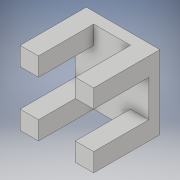
# Autodesk Inventor part: STand_1
Saved by Autodesk Inventor 2019 (Build 230136000, 136)
## iProperties
Created: 2020-02-20
Part Number: STand_1
Material: Generic
Document SubType Name: Modeling
Designer: Chirag
Density: 1 g/cm^3
Appearance: Default
Author: Chirag
Autodesk Inventor part; units mm, degrees
ref_plane "YZ Plane" through (0, 0, 0) normal (1, 0, 0) x (0, 1, 0)
ref_plane "XZ Plane" through (0, 0, 0) normal (0, 1, 0) x (-1, 0, 0)
ref_plane "XY Plane" through (0, 0, 0) normal (0, 0, 1) x (1, 0, 0)
sketch "Sketch1" plane through (0, 0, 0) normal (0, 0, 1) x (1, 0, 0)
  line L0 (0, 0) -> (0, -200)
  line L1 (0, -200) -> (200, -200)
  line L2 (200, -200) -> (200, 0)
  line L3 (200, 0) -> (0, 0)
  dimension "d0" = 200
  dimension "d1" = 200
  constraints: 8 end point, 2 parallel, 1 perpendicular, 1 vertical
  measures "d0" distance of L0.start L0.end
  measures "d1" distance of L1.end L0.end
extrude "Extrusion1" add sketch "Sketch1" along normal blind 30
sketch "Sketch2" plane through (0, 0, 30) normal (0, 0, 1) x (1, 0, 0)
  line L0 (0, 0) -> (0, -200) projected
  line L1 (0, 0) -> (0, -50)
  line L2 (0, -50) -> (50, -50)
  line L3 (50, -50) -> (50, 0)
  line L4 (50, 0) -> (0, 0)
  line L5 (200, -200) -> (200, 0) projected
  line L6 (200, 0) -> (200, -50)
  line L7 (200, -50) -> (150, -50)
  line L8 (150, -50) -> (150, 0)
  line L9 (150, 0) -> (200, 0)
  line L10 (0, -200) -> (0, -150)
  line L11 (0, -150) -> (50, -150)
  line L12 (50, -150) -> (50, -200)
  line L13 (50, -200) -> (0, -200)
  line L14 (200, -200) -> (200, -150)
  line L15 (200, -150) -> (150, -150)
  line L16 (150, -150) -> (150, -200)
  line L17 (150, -200) -> (200, -200)
  dimension "d4" = 50
  dimension "d5" = 50
  dimension "d6" = 50
  dimension "d7" = 50
  dimension "d8" = 50
  dimension "d9" = 50
  dimension "d10" = 50
  dimension "d11" = 50
  constraints: 32 end point, 8 parallel, 4 perpendicular, 4 point on line
  measures "d4" distance of L0.start L1.end
  measures "d5" distance of L2.end L1.end
  measures "d6" distance of L5.end L6.end
  measures "d7" distance of L6.end L7.end
  measures "d8" distance of L0.end L10.end
  measures "d9" distance of L10.end L11.end
  measures "d10" distance of L5.start L14.end
  measures "d11" distance of L15.end L14.end
extrude "Extrusion2" add sketch "Sketch2" along normal blind 150
body "Solid1"
